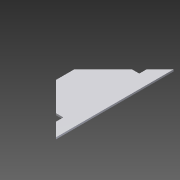
# Autodesk Inventor part: top short
Saved by Autodesk Inventor 2015 (Build 190159000, 159)
## iProperties
Created: 2019-04-10
Part Number: top short
Material: Generic
Document SubType Name: Modeling
Designer: Raptor
Density: 1 g/cm^3
Appearance: Snow
Author: Raptor
Autodesk Inventor part; units mm, degrees
ref_plane "YZ Plane" through (0, 0, 0) normal (1, 0, 0) x (0, 1, 0)
ref_plane "XZ Plane" through (0, 0, 0) normal (0, 1, 0) x (-1, 0, 0)
ref_plane "XY Plane" through (0, 0, 0) normal (0, 0, 1) x (1, 0, 0)
sketch "Sketch1" plane through (0, 0, 0) normal (0, 1, 0) x (-1, 0, 0)
  line L0 (0, 0) -> (0, -1300)
  line L1 (550, -750) -> (550, -550)
  line L2 (150, -150) -> (150, -230)
  line L3 (150, -230) -> (230, -230)
  line L4 (0, 0) -> (150, -150)
  line L5 (230, -230) -> (550, -550)
  line L6 (150, -1150) -> (150, -1070)
  line L7 (150, -1070) -> (230, -1070)
  line L8 (0, -1300) -> (150, -1150)
  line L9 (230, -1070) -> (550, -750)
  dimension "d3" = 1300
  dimension "d6" = 550
  dimension "d7" = 150
  dimension "d8" = 80
  dimension "d9" = 45
  dimension "d10" = 80
  dimension "d11" = 150
  dimension "d12" = 45
  constraints: 20 end point, 3 vertical, 2 collinear, 2 perpendicular, 1 parallel
  measures "d3" distance of L0.start L0.end
  measures "d6" distance between parallel lines of L0 L1
  measures "d7" distance between parallel lines of L0 L2
  measures "d8" distance of L2.start L2.end
  measures "d9" angle of L4 L0
  measures "d10" distance of L6.start L6.end
  measures "d11" distance between parallel lines of L0 L6
  measures "d12" angle of L0 L8
extrude "Extrusion1" add sketch "Sketch1" along normal blind 20
fillet "Fillet1" radius 5 1 edges at (-150, 10, -230)
fillet "Fillet2" radius 5 1 edges at (-150, 10, -1070)
body "Solid1"
